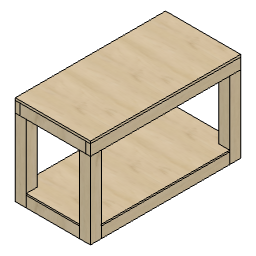
workbench_v1.4 (Autodesk Fusion 360 design; units mm, degrees)
Autodesk Fusion 360 part; units mm, degrees
note: some values were not read from the file. Set by a fixed rule: which face or edge a step refers to.
sketch "Sketch1" plane through (0, 0, 0) normal (0, 0, 1) x (1, 0, 0)
  line L0 (0, 0) -> (38.1, 0)
  line L1 (38.1, 0) -> (38.1, 88.9)
  line L2 (38.1, 88.9) -> (0, 88.9)
  line L3 (0, 88.9) -> (0, 0)
  dimension "d6" = 38.1
  dimension "d7" = 88.9
  constraint horizontal L0
  constraint vertical L1
  constraint horizontal L2
  constraint vertical L3
  constraint coincident L0.start L3.end
  measures "d6" distance of L0.start L0.end
  measures "d7" distance of L0.start L2.end
extrude "Extrude1" add sketch "Sketch1" along normal blind 1219.2 makes body 1
copy_body "CopyPasteBodies1" bodies 1 makes body 2
move_body "Move1" bodies 2 to x (1, 0, 0) y (0, 1, 0) z (0, 0, 1) at (368.3, 0, 0)
sketch "Sketch2" plane through (0, 0, 0) normal (0, 1, 0) x (1, 0, 0)
  line L0 (-101.6, 0) -> (508, 0)
  line L1 (508, 0) -> (508, -1219.2)
  line L2 (508, -1219.2) -> (-101.6, -1219.2)
  line L3 (-101.6, -1219.2) -> (-101.6, 0)
  dimension "d11" = 609.6
  dimension "d12" = 1219.2
  constraint horizontal L0
  constraint vertical L1
  constraint horizontal L2
  constraint vertical L3
  measures "d11" distance of L0.start L0.end
  measures "d12" distance of L0.start L2.end
extrude "Extrude2" add sketch "Sketch2" along normal blind 19.05 separate body makes body 3
move_body "Move2" bodies 3 to x (1, 0, 0) y (0, 1, 0) z (0, 0, 1) at (0, 88.9, 0)
sketch "Sketch3" plane through (0, 88.9, 0) normal (0, -1, 0) x (1, 0, 0)
  line L0 (508, 1219.2) -> (-101.6, 1219.2)
  line L1 (-101.6, 1219.2) -> (-101.6, 0)
  line L2 (-101.6, 0) -> (508, 0)
  line L3 (508, 0) -> (508, 1219.2)
  line L4 (-101.6, 101.6) -> (508, 101.6)
  line L5 (508, 101.6) -> (508, 139.7)
  line L6 (508, 139.7) -> (-101.6, 139.7)
  line L7 (-101.6, 139.7) -> (-101.6, 101.6)
  dimension "d16" = 609.6
  dimension "d17" = 38.1
  constraint horizontal L4
  constraint vertical L5
  constraint horizontal L6
  constraint vertical L7
  constraint coincident L1 L4.start
  measures "d16" distance of L4.start L4.end
  measures "d17" distance of L4.start L6.end
extrude "Extrude3" add sketch "Sketch3" along normal blind 88.9 separate body contours L1 L3 L4 L5 L6 L7 makes body 4
copy_body "CopyPasteBodies2" bodies 4 makes body 5
move_body "Move3" bodies 5 to x (1, 0, 0) y (0, 1, 0) z (0, 0, 1) at (0, 0, 977.9)
copy_body "CopyPasteBodies3" bodies 5 makes body 6
move_body "Move4" bodies 6 to x (1, 0, 0) y (0, 1, 0) z (0, 0, 1) at (0, 0, -508)
move_body "Move5" bodies 6 to x (1, 0, 0) y (0, 1, 0) z (0, 0, 1) at (0, 0, 38.1)
move_body "Move6" bodies 6 to x (1, 0, 0) y (0, 1, 0) z (0, 0, 1) at (0, 0, -19.05)
sketch "Sketch4" plane through (0, 88.9, 0) normal (0, -1, 0) x (1, 0, 0)
  line L0 (508, 1219.2) -> (-101.6, 1219.2)
  line L1 (-101.6, 1219.2) -> (-101.6, 0)
  line L2 (-101.6, 0) -> (508, 0)
  line L3 (508, 0) -> (508, 1219.2)
  line L4 (38.1, 1117.6) -> (76.2, 1117.6)
  line L5 (76.2, 1117.6) -> (76.2, 1028.7)
  line L6 (76.2, 1028.7) -> (38.1, 1028.7)
  line L7 (38.1, 1028.7) -> (38.1, 1117.6)
  dimension "d20" = 38.1
  dimension "d21" = 88.9
  constraint horizontal L4
  constraint vertical L5
  constraint horizontal L6
  constraint vertical L7
  measures "d20" distance of L4.start L4.end
  measures "d21" distance of L4.start L6.end
extrude "Extrude4" add sketch "Sketch4" along normal blind 622.3 separate body contours L4 L5 L6 L7 makes body 7
move_body "Move7" bodies 7 to x (1, 0, 0) y (0, 1, 0) z (0, 0, 1) at (-76.2, 0, 0)
copy_body "CopyPasteBodies4" bodies 7 makes body 8
move_body "Move8" bodies 8 to x (1, 0, 0) y (0, 1, 0) z (0, 0, 1) at (444.5, 0, 0)
copy_body "CopyPasteBodies5" bodies 8 7 makes body 9 makes body 10
move_body "Move9" bodies 9 10 to x (1, 0, 0) y (0, 1, 0) z (0, 0, 1) at (0, 0, -927.1)
move_body "Move10" bodies 7 to x (0, 0, 1) y (0, 1, 0) z (-1, 0, 0) at (1117.6, 0, 1079.5)
move_body "Move11" bodies 8 to x (0, 0, 1) y (0, 1, 0) z (-1, 0, 0) at (1435.1, 0, 635)
move_body "Move12" bodies 9 to x (0, 0, 1) y (0, 1, 0) z (-1, 0, 0) at (508, 0, -266.7)
move_body "Move13" bodies 10 to x (0, 0, 1) y (0, 1, 0) z (-1, 0, 0) at (139.7, 0, 177.8)
move_body "Move14" bodies 10 to x (1, 0, 0) y (0, 1, 0) z (0, 0, 1) at (50.8, 0, 0)
copy_body "CopyPasteBodies6" bodies 1 2 4 5 6 makes body 11 makes body 12 makes body 13 makes body 14 makes body 15
move_body "Move15" bodies 11 12 13 14 15 to x (1, 0, 0) y (0, 1, 0) z (0, 0, 1) at (0, -622.3, 0)
split "Split1" by plane through (406.4, -622.3, 0) normal (1, 0, 0) bodies 15 14 13 makes body 18 at (440.2667, -563.0333, 101.6) makes body 17 at (440.2667, -563.0333, 1079.5) makes body 16 at (440.2667, -563.0333, 590.55)
delete_body "RemoveBody1" bodies 18
delete_body "RemoveBody2" bodies 17
delete_body "RemoveBody3" bodies 16
split "Split2" by plane through (0, -533.4, 0) normal (-1, 0, 0) bodies 13 15 14 makes body 21 at (-67.7333, -563.0333, 1079.5) makes body 20 at (-67.7333, -563.0333, 590.55) makes body 19 at (-67.7333, -563.0333, 101.6)
delete_body "RemoveBody4" bodies 19
delete_body "RemoveBody5" bodies 20
delete_body "RemoveBody6" bodies 21
move_body "Move16" bodies 13 to x (1, 0, 0) y (0, 1, 0) z (0, 0, 1) at (0, 0, 76.2)
move_body "Move17" bodies 14 to x (1, 0, 0) y (0, 1, 0) z (0, 0, 1) at (0, 0, -76.2)
split "Split3" by plane through (406.4, 88.9, 139.7) normal (0, 0, -1) bodies 12 11 makes body 23 at (0, -563.0333, 46.5667) makes body 22 at (368.3, -563.0333, 93.1333)
delete_body "RemoveBody7" bodies 22
delete_body "RemoveBody8" bodies 23
split "Split4" by plane through (317.5, 88.9, 1079.5) normal (0, 0, 1) bodies 12 11 makes body 25 at (0, -563.0333, 1172.6333) makes body 24 at (368.3, -563.0333, 1172.6333)
delete_body "RemoveBody9" bodies 24
delete_body "RemoveBody10" bodies 25
sketch "Sketch5" plane through (0, -533.4, 0) normal (0, 1, 0) x (-1, 0, 0)
  line L0 (0, 215.9) -> (-406.4, 215.9)
  line L1 (-406.4, 215.9) -> (-406.4, 177.8)
  line L2 (-406.4, 177.8) -> (0, 177.8)
  line L3 (0, 177.8) -> (-406.4, 177.8)
  line L4 (-406.4, 177.8) -> (-406.4, 1041.4)
  line L5 (-406.4, 1041.4) -> (0, 1041.4)
  line L6 (0, 1041.4) -> (0, 177.8)
  line L7 (0, 177.8) -> (0, 215.9)
  dimension "d25" = 406.4
  dimension "d26" = 863.6
  constraint horizontal L3
  constraint vertical L4
  constraint horizontal L5
  constraint vertical L6
  constraint coincident L2.end L3.start
  measures "d25" distance of L2.end L1.end
  measures "d26" distance of L2.end L5.end
extrude "Extrude5" add sketch "Sketch5" along normal blind 12.7 separate body makes body 26
move_body "Move18" bodies 7 8 to x (1, 0, 0) y (0, 1, 0) z (0, 0, 1) at (0, 0, 139.7)
move_body "Move19" bodies 9 10 to x (1, 0, 0) y (0, 1, 0) z (0, 0, 1) at (0, 0, -139.7)
move_body "Move20" bodies 8 9 to x (1, 0, 0) y (0, 1, 0) z (0, 0, 1) at (101.6, 0, 0)
move_body "Move21" bodies 10 7 to x (1, 0, 0) y (0, 1, 0) z (0, 0, 1) at (-101.6, 0, 0)
move_face "OffsetFaces1" offset 50.8 2 faces at (478.3667, -118.5333, 1181.1) (-42.3333, -118.5333, 1181.1) on bodies 7 8
move_face "OffsetFaces2" offset 50.8 2 faces at (448.7333, -118.5333, 38.1) (-71.9667, -118.5333, 38.1) on bodies 9 10
move_body "Move22" bodies 7 10 9 8 to x (1, 0, 0) y (0, 1, 0) z (0, 0, 1) at (0, -88.9, 0)
move_body "Move23" bodies 11 to x (1, 0, 0) y (0, 1, 0) z (0, 0, 1) at (-101.6, 0, 0)
move_body "Move24" bodies 12 to x (1, 0, 0) y (0, 1, 0) z (0, 0, 1) at (101.6, 0, 0)
move_body "Move25" bodies 13 to x (1, 0, 0) y (0, 1, 0) z (0, 0, 1) at (0, 0, -177.8)
move_body "Move26" bodies 14 to x (1, 0, 0) y (0, 1, 0) z (0, 0, 1) at (0, 0, 177.8)
move_body "Move27" bodies 1 to x (1, 0, 0) y (0, 1, 0) z (0, 0, 1) at (-101.6, 0, 0)
move_body "Move28" bodies 2 to x (1, 0, 0) y (0, 1, 0) z (0, 0, 1) at (101.6, 0, 0)
move_body "Move29" bodies 4 to x (1, 0, 0) y (0, 1, 0) z (0, 0, 1) at (0, 0, -101.6)
move_body "Move30" bodies 5 to x (1, 0, 0) y (0, 1, 0) z (0, 0, 1) at (0, 0, 101.6)
move_face "OffsetFaces3" offset -38.1 3 faces at (-101.6, 59.2667, 615.95) (-101.6, 59.2667, 25.4) (-101.6, 59.2667, 1206.5) on bodies 4 5 6
move_face "OffsetFaces4" offset -38.1 3 faces at (508, 29.6333, 603.25) (508, 29.6333, 12.7) (508, 29.6333, 1193.8) on bodies 4 5 6
move_face "OffsetFaces5" offset 50.8 2 faces at (-88.9, -592.6667, 139.7) (482.6, -592.6667, 139.7) on bodies 11 12
move_face "OffsetFaces6" offset 50.8 2 faces at (-88.9, -563.0333, 1079.5) (482.6, -563.0333, 1079.5) on bodies 11 12
move_face "OffsetFaces7" offset 12.7 2 faces at (0, -563.0333, 1193.8) (0, -563.0333, 12.7) on bodies 13 14
move_face "OffsetFaces8" offset 12.7 2 faces at (406.4, -592.6667, 1193.8) (406.4, -592.6667, 12.7) on bodies 13 14
move_face "OffsetFaces9" offset 63.5 1 faces at (406.4, -592.6667, 603.25) on bodies 15
move_face "OffsetFaces10" offset 63.5 1 faces at (0, -563.0333, 603.25) on bodies 15
move_face "OffsetFaces11" offset 177.8 1 faces at (270.9333, -529.1667, 1041.4) on bodies 26
move_face "OffsetFaces12" offset 177.8 1 faces at (270.9333, -529.1667, 177.8) on bodies 26
move_face "OffsetFaces13" offset 12.7 2 faces at (0, -529.1667, 143.9333) (0, -524.9333, 550.3333) on bodies 26
move_face "OffsetFaces14" offset 12.7 2 faces at (406.4, -524.9333, 71.9667) (406.4, -524.9333, 550.3333) on bodies 26
sketch "Sketch6" plane through (419.1, 0, 0) normal (1, 0, 0) x (0, 0, -1)
  line L0 (-1219.2, -533.4) -> (0, -533.4)
  line L1 (0, -533.4) -> (0, -520.7)
  line L2 (0, -520.7) -> (-1219.2, -520.7)
  line L3 (-1219.2, -520.7) -> (-1219.2, -533.4)
  line L4 (-1130.7571, -533.4) -> (-89.3571, -533.4)
  line L5 (-89.3571, -533.4) -> (-89.3571, -520.7)
  line L6 (-89.3571, -520.7) -> (-1130.7571, -520.7)
  line L7 (-1130.7571, -520.7) -> (-1130.7571, -533.4)
  dimension "d43" = 1041.4
  dimension "d44" = 12.7
  constraint horizontal L4
  constraint vertical L5
  constraint horizontal L6
  constraint vertical L7
  constraint coincident L0 L4.start
  measures "d43" distance of L4.start L4.end
  measures "d44" distance of L4.start L6.end
extrude "Extrude6" add sketch "Sketch6" along normal blind 88.9 contours L0 L2 L4 L5 L6 L7 bodies 26
sketch "Sketch7" plane through (-12.7, 0, 0) normal (-1, 0, 0) x (0, 0, 1)
  line L0 (0, -533.4) -> (1219.2, -533.4)
  line L1 (1219.2, -533.4) -> (1219.2, -520.7)
  line L2 (1219.2, -520.7) -> (0, -520.7)
  line L3 (0, -520.7) -> (0, -533.4)
  line L4 (88.9023, -533.4) -> (1130.3023, -533.4)
  line L5 (1130.3023, -533.4) -> (1130.3023, -520.7)
  line L6 (1130.3023, -520.7) -> (88.9023, -520.7)
  line L7 (88.9023, -520.7) -> (88.9023, -533.4)
  dimension "d47" = 1041.4
  dimension "d48" = 12.7
  constraint horizontal L4
  constraint vertical L5
  constraint horizontal L6
  constraint vertical L7
  constraint coincident L0 L4.start
  measures "d47" distance of L4.start L4.end
  measures "d48" distance of L4.start L6.end
extrude "Extrude7" add sketch "Sketch7" along normal blind 88.9 contours L0 L2 L4 L5 L6 L7 bodies 26
equation "woodWidth = 1.5 in"
equation "woodHeight = 3.5 in"
equation "benchHeight = 24.5 in"
equation "benchWidth = 48 in"
equation "benchDepth = 24 in"
equation "d6 = woodWidth"
equation "d7 = woodHeight"
equation "d8 = benchWidth"
equation "insets = 4 in"
equation "d11 = benchDepth"
equation "d12 = benchWidth"
equation "tableTopHeight = 0.75 in"
equation "d14 = tableTopHeight"
equation "d16 = benchDepth"
equation "d17 = woodWidth"
equation "d18 = woodHeight"
equation "d20 = woodWidth"
equation "d21 = woodHeight"
equation "d22 = benchHeight"
equation "shelfTopHeight = 0.5 in"
equation "d25 = benchDepth - insets * 2"
equation "d26 = benchWidth - insets * 2 - woodWidth * 4"
equation "d27 = shelfTopHeight"
named bodies: "Top Rail 1", "Top Rail 2", "Table Top", "Top Rib 1", "Top Rib 2", "Top Rib 3", "Leg 1", "Leg 2", "Leg 3", "Leg 4", "Top Rib 1 (1)", "Top Rib 2 (1)", "Bottom Rail 1", "Bottom Rail 2", "Bottom Rib 1", "Bottom Rib 2", "Bottom Rib 3", "Bottom Rib 3 (1)", "Bottom Rib 2 (1)", "Bottom Rib 1 (1)", "Bottom Rail 2 (1)", "Bottom Rail 1 (1)", "Shelf Top"
